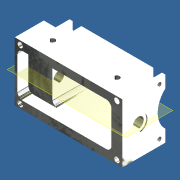
# Autodesk Inventor part: CarterRouleau
Saved by Autodesk Inventor 2018 (Build 220112000, 112)
## iProperties
Created: 2022-04-28
Part Number: CarterRouleau
Material: Aluminum 6061
Document SubType Name: Modeling
Designer: Nathann
Density: 2.7 g/cm^3
Appearance: Aluminum - Flat
Mass: 243.703 g
Surface Area: 289.798 cm^2
Volume: 90.2603 cm^3
Author: Nathann
Autodesk Inventor part; units mm, degrees
ref_plane "YZ Plane" through (0, 0, 0) normal (1, 0, 0) x (0, 1, 0)
ref_plane "XZ Plane" through (0, 0, 0) normal (0, 1, 0) x (-1, 0, 0)
sketch "Sketch1" plane through (0, 0, 0) normal (0, 1, 0) x (-1, 0, 0)
  line L0 (0, 0) -> (100, 0)
  line L1 (100, 0) -> (100, 55)
  line L2 (100, 55) -> (0, 55)
  line L3 (0, 55) -> (0, 0)
  dimension "d0" = 55
  dimension "d1" = 100
  constraints: 8 end point, 2 parallel, 1 horizontal, 1 perpendicular
  measures "d0" distance of L0.end L1.end
  measures "d1" distance of L1.end L2.end
extrude "Extrusion1" add sketch "Sketch1" along normal blind 40
sketch "Sketch2" plane through (0, 0, 0) normal (0, -1, 0) x (1, 0, 0)
  circle A0 centre (-5, 3.75) radius 2.5
  line L0 (0, 55) -> (0, 0) projected
  line L1 (0, 0) -> (-100, 0) projected
  line L2 (0, 0) -> (-100, 0) projected
  line L3 (-50, 0) -> (-50, 13.5836)
  line L4 (0, 55) -> (0, 0) projected
  line L5 (0, 27.5) -> (-21.4459, 27.5)
  circle A1 centre (-5, 51.25) radius 2.5
  circle A2 centre (-95, 3.75) radius 2.5
  circle A3 centre (-95, 51.25) radius 2.5
  dimension "d4" = 5
  dimension "d5" = 5
  dimension "d6" = 3.75
  constraints: 4 centre point, 4 end point, 3 symmetric about line, 2 midpoint, 1 horizontal, 1 vertical, 3 other
  measures "d4" distance from line of L0 A0.centre
  measures "d5" diameter of A0
  measures "d6" distance from line of L1 A0.centre
extrude "Extrusion2" cut sketch "Sketch2" against normal blind 18
sketch "Sketch3" plane through (0, 0, 0) normal (0, -1, 0) x (1, 0, 0)
  line L0 (-97.5, 7.5) -> (-10, 7.5)
  line L1 (-10, 7.5) -> (-10, 47.5)
  line L2 (-10, 47.5) -> (-97.5, 47.5)
  line L3 (-97.5, 47.5) -> (-97.5, 7.5)
  line L4 (-100, 0) -> (-100, 55) projected
  line L5 (-100, 55) -> (0, 55) projected
  point P0 (0, 0)
  dimension "d9" = 2.5
  dimension "d10" = 87.5
  dimension "d11" = 40
  dimension "d12" = 55
  dimension "d13" = 7.5
  constraints: 8 end point, 2 parallel, 1 horizontal, 1 perpendicular
  measures "d9" distance between parallel lines of L4 L3
  measures "d10" distance of L1.end L2.end
  measures "d11" distance of L2.end L0.start
  measures "d12" distance of L4.start L4.end
  measures "d13" distance between parallel lines of L5 L2
extrude "Extrusion3" cut sketch "Sketch3" against normal blind 10
sketch "Sketch4" plane through (0, 10, 0) normal (0, -1, 0) x (1, 0, 0)
  line L0 (-10, 47.5) -> (-10, 7.5) projected
  line L1 (-97.5, 47.5) -> (-10, 47.5) projected
  line L2 (-10, 7.5) -> (-75, 7.5)
  line L3 (-75, 7.5) -> (-75, 47.5)
  line L4 (-75, 47.5) -> (-10, 47.5)
  line L5 (-10, 47.5) -> (-10, 7.5)
  point P0 (0, 0)
  dimension "d16" = 65
  constraints: 8 end point, 2 parallel, 1 horizontal, 1 perpendicular, 1 point on line
  measures "d16" distance between parallel lines of L0 L3
extrude "Extrusion4" cut sketch "Sketch4" against normal through all
sketch "Sketch5" plane through (0, 0, 55) normal (1, 0, 0) x (0, 0, -1)
  circle A0 centre (27.5, 16) radius 5
  line L0 (55, 0) -> (55, 40) projected
  line L1 (0, 0) -> (0, 40) projected
  line L2 (0, 0) -> (55, 0) projected
  dimension "d19" = 27.5
  dimension "d20" = 55
  dimension "d21" = 10
  dimension "d22" = 16
  constraints: 1 centre point
  measures "d19" distance from line of L0 A0.centre
  measures "d20" distance between parallel lines of L1 L0
  measures "d21" diameter of A0
  measures "d22" distance from line of L2 A0.centre
extrude "Extrusion5" cut sketch "Sketch5" against normal through all
sketch "Sketch6" plane through (0, 0, 55) normal (1, 0, 0) x (0, 0, -1)
  circle A0 centre (27.5, 16) radius 5 projected
  circle A1 centre (27.5, 16) radius 7.5
  point P0 (55, 0)
  dimension "d25" = 15
  constraints: 1 centre point, 1 coincident
  measures "d25" diameter of A1
extrude "Extrusion6" cut sketch "Sketch6" against normal blind 1
sketch "Sketch7" plane through (-100, 0, 0) normal (-1, 0, 0) x (0, 0, 1)
  circle A0 centre (27.5, 16) radius 5 projected
  circle A1 centre (27.5, 16) radius 7.5
  point P0 (0, 0)
  dimension "d28" = 15
  constraints: 1 centre point, 1 coincident
  measures "d28" diameter of A1
extrude "Extrusion7" cut sketch "Sketch7" against normal blind 1
sketch "Sketch8" plane through (-100, 0, 55) normal (0, 0, 1) x (1, 0, 0)
  circle A0 centre (80, 15) radius 2.5
  line L0 (100, 0) -> (100, 40) projected
  line L1 (0, 0) -> (100, 0) projected
  circle A1 centre (20, 15) radius 2.5
  line L2 (0, 0) -> (0, 40) projected
  dimension "d31" = 5
  dimension "d32" = 20
  dimension "d33" = 15
  dimension "d34" = 5
  dimension "d35" = 20
  dimension "d36" = 15
  constraints: 2 centre point
  measures "d31" diameter of A0
  measures "d32" distance from line of L0 A0.centre
  measures "d33" distance from line of L1 A0.centre
  measures "d34" diameter of A1
  measures "d35" distance from line of L2 A1.centre
  measures "d36" distance from line of L1 A1.centre
extrude "Extrusion8" cut sketch "Sketch8" against normal blind 15
ref_plane "Work Plane1" through (-100, 0, 27.5) normal (0, 0, 1) x (1, 0, 0)
mirror "Mirror1" about plane through (-100, 0, 27.5) normal (0, 0, 1) of "Extrusion8"
fillet "Fillet1" radius 5 6 edges at (-97.5, 5, 7.5) (-97.5, 5, 47.5) (-10, 20, 7.5) (-10, 20, 47.5) (-75, 25, 7.5) (-75, 25, 47.5)
sketch "Sketch10" plane through (0, 40, 0) normal (0, 1, 0) x (1, 0, 0)
  arc A0 (-78, -48) -> (-86, -48) centre (-82, -48) ccw
  line L0 (-78, -48) -> (-78, -67.7659)
  line L1 (-78, -67.7659) -> (-86, -67.7659)
  line L2 (-86, -67.7659) -> (-86, -48)
  line L3 (-100, -55) -> (0, -55) projected
  line L4 (-100, 0) -> (-100, -55) projected
  arc A1 (-3, -48) -> (-11, -48) centre (-7, -48) ccw
  line L5 (-3, -48) -> (-3, -67.2517)
  line L6 (-3, -67.2517) -> (-11, -67.2517)
  line L7 (-11, -67.2517) -> (-11, -48)
  line L8 (0, -55) -> (0, 0) projected
  line L9 (-100, 0) -> (-100, -55) projected
  line L10 (-100, -27.5) -> (-88.5894, -27.5)
  arc A2 (-86, -7) -> (-78, -7) centre (-82, -7) ccw
  line L11 (-78, -7) -> (-78, 12.7659)
  line L12 (-78, 12.7659) -> (-86, 12.7659)
  line L13 (-86, 12.7659) -> (-86, -7)
  line L14 (-100, 0) -> (0, 0)
  arc A3 (-11, -7) -> (-3, -7) centre (-7, -7) ccw
  line L15 (-3, -7) -> (-3, 12.2517)
  line L16 (-3, 12.2517) -> (-11, 12.2517)
  line L17 (-11, 12.2517) -> (-11, -7)
  dimension "d40" = 8
  dimension "d41" = 7
  dimension "d43" = 8
  dimension "d44" = 7
  dimension "d45" = 7
  dimension "d48" = 82
  constraints: 28 end point, 10 symmetric about line, 8 point on circle, 4 centre point, 2 parallel, 1 horizontal, 1 midpoint, 2 other
  measures "d40" diameter of A0
  measures "d41" distance from line of L3 A0.centre
  measures "d43" diameter of A1
  measures "d44" distance from line of A1.centre L8
  measures "d45" distance from line of L3 A1.centre
  measures "d48" distance from line of L8 A0.centre
extrude "Extrusion9" cut sketch "Sketch10" against normal blind 8 contours L0 L3 L2 A0 | L0 L1 L2 L3 | L7 A1 L5 L3 | L3 L5 L6 L7 | L14 L11 A2 L13 | L13 L12 L11 L14 | L15 A3 L17 L14 | L14 L17 L16 L15
sketch "Sketch11" plane through (0, 0, 0) normal (-1, 0, 0) x (0, 0, 1)
  circle A0 centre (5.5, 34.5) radius 2
  line L0 (0, 40) -> (55, 40) projected
  line L1 (0, 0) -> (0, 40) projected
  line L2 (55, 40) -> (0, 40) projected
  line L3 (27.5, 40) -> (27.5, 46.5712)
  circle A1 centre (49.5, 34.5) radius 2
  dimension "d49" = 4
  dimension "d50" = 5.5
  dimension "d51" = 5.5
  constraints: 2 centre point, 2 end point, 1 midpoint, 1 symmetric about line, 1 vertical, 1 other
  measures "d49" diameter of A0
  measures "d50" distance from line of L0 A0.centre
  measures "d51" distance from line of L1 A0.centre
extrude "Extrusion10" cut sketch "Sketch11" along normal blind 13
sketch "Sketch12" plane through (0, 40, 0) normal (0, 1, 0) x (1, 0, 0)
  line L0 (-100, -55) -> (0, -55) projected
  line L1 (0, 0) -> (-100, 0) projected
  line L2 (-100, -55) -> (-89, -55)
  line L3 (-89, -55) -> (-89, 0)
  line L4 (-89, 0) -> (-100, 0)
  line L5 (-100, 0) -> (-100, -55)
  line L6 (-86, -55) -> (-86, -48) projected
  dimension "d54" = 3
  constraints: 8 end point, 2 parallel, 1 horizontal, 1 perpendicular, 1 point on line
  measures "d54" distance between parallel lines of L6 L3
extrude "Extrusion11" cut sketch "Sketch12" against normal blind 13
sketch "Sketch13" plane through (-89, 40, 0) normal (-1, 0, 0) x (0, 0, 1)
  circle A0 centre (5.5, -5.5) radius 2 projected
  circle A1 centre (49.5, -5.5) radius 2 projected
  point P0 (0, -40)
extrude "Extrusion12" cut sketch "Sketch13" against normal blind 13
sketch "Sketch15" plane through (-89, 40, 0) normal (-1, 0, 0) x (0, 0, 1)
  circle A0 centre (27.5, 15) radius 22
  line L0 (0, -13) -> (0, 0) projected
  line L1 (0, 0) -> (55, 0) projected
  point P0 (0, -40)
  dimension "d59" = 27.5
  dimension "d60" = 15
  dimension "d61" = 44
  constraints: 1 centre point
  measures "d59" distance from line of A0.centre L0
  measures "d60" distance from line of L1 A0.centre
  measures "d61" diameter of A0
extrude "Extrusion13" cut sketch "Sketch15" against normal through all
equation "\"d13\" = -0.5 * d11 + 0.5 * d12"
equation "\"d19\" = 0.5 * d20"
equation "\"d36\" = d33"
equation "\"d51\" = d50"
body "Solid1"
